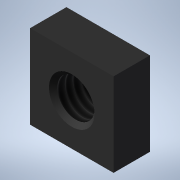
# Autodesk Inventor part: HNSQ3-3
Saved by Autodesk Inventor 2021 (Build 250183000, 183)
## iProperties
Category: PARTsolutions
Company: MISUMI
Created: 2024-12-13
Part Number: HNSQ3-3
Material: Generic
Catalog Web Link: www.cadenas.de
Description: HNSQ-Square Nuts for Aluminum Frame - 15mm Square
Vendor: MISUMI
Document SubType Name: Modeling
Designer: psAdmin
Manufacturer: MISUMI
Mass: 0.0605956 g
Surface Area: 1.20085 cm^2
Volume: 0.0605956 cm^3
Density: 1 g/cm^3
Appearance: PSOLRGB-175-175-175
PSOL_IDENT_0: {$CADENAS_DATA/23d-libs/misumi/metric/38_al_extrusions_blackets/hnsq.prj},153 {VTYP=3D},{NB=HNSQ3-3}
PSOL_IDENT_1: ,{LINA=HNSQ3-3},{NN=HNSQ},{DATE=30.06.2021 13:17:54},{GEOMDATE=23.09.2009 05:53:00},{VERSION=},{LINE
PSOL_IDENT_2: ID=270},{WBVAR=},{WBNUMERIC=}  {NB=HNSQ3-3},{LINA=HNSQ3-3},{KT=DUMMY},{PN=HNSQ3-3},{TYPE=HNSQ},{MAT=
PSOL_IDENT_3: SS400(1018 Steel Equivalent)(1.0040_Ust.42.2)},{ST=Trivalent Chromate},{NO=3},{M=3},{AF=HFS3-1515}
NB: HNSQ3-3
NN: HNSQ
NT: Square Nuts for Aluminum Frame - 15mm Square
NBSYN: $PN.
LINA: HNSQ3-3
CATALOG: Misumi
PN: HNSQ3-3
MAT: SS400(1018 Steel Equivalent)(1.0040_Ust.42.2)
ST: Trivalent Chromate Plating
NO: 3
M: 3
AF: HFS3-1515
SUPPLIER: MISUMI
ARTICLENO: HNSQ3-3
BOMINFO: HNSQ3-3
CREATOR: CADENAS GmbH
Title: HNSQ3-3
Author: Cadenas PARTsolutions
Comments: Square Nuts for Aluminum Frame - 15mm Square
Autodesk Inventor part; units mm, degrees
sketch "Sketch_1" plane through (0, 0, 0) normal (0, 0, 1) x (1, 0, 0)
  line L0 (-2.75, -2.75) -> (2.75, -2.75)
  line L1 (2.75, -2.75) -> (2.75, 2.75)
  line L2 (2.75, 2.75) -> (-2.75, 2.75)
  line L3 (-2.75, 2.75) -> (-2.75, -2.75)
  constraints: 8 end point
extrude "Extrusion1" add sketch "Sketch_1" along normal mid plane 2.4
sketch "Sketch_2" plane through (0, 0, 0) normal (0, 1, 0) x (-1, 0, 0)
  line L0 (0, 1.2) -> (0, -1.2)
  line L1 (0, -1.2) -> (-1.5, -1.2)
  line L2 (-1.5, -1.2) -> (-1.2295, -0.9295)
  line L3 (-1.2295, -0.9295) -> (-1.2295, 0.9295)
  line L4 (-1.2295, 0.9295) -> (-1.5, 1.2)
  line L5 (-1.5, 1.2) -> (0, 1.2)
  line L6 (0, 1.2) -> (0, -1.2)
  constraints: 14 end point
revolve "Revolution1" cut sketch "Sketch_2" angle 360 about axis through (0, 0, 1.2) along (0, 0, 1)
thread "Thread1" size "M3x0.5" class "6H" standard "ISO Metric profile" full length
ref_plane "nut_to_bolt_XY" through (0, 0, -1.2) normal (0, 0, 1) x (1, 0, 0)
ref_plane "nut_to_bolt_YZ" through (0, 0, -1.2) normal (1, 0, 0) x (0, 1, 0)
ref_plane "nut_to_bolt_ZX" through (0, 0, -1.2) normal (0, 1, 0) x (0, 0, 1)
body "Solid1"
